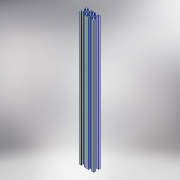
# Autodesk Inventor part: Profile horizontal 20x40x360
Saved by Autodesk Inventor 2017 (Build 210142000, 142)
## iProperties
Company: FABLAB Frenchmakers
Part Number: Profile horizontal 20x40x360
Material: Aluminium
Document SubType Name: Modeling
Designer: FABLAB Frenchmakers
Density: 2.7 g/cm^3
Appearance: Aluminium - Plat(2)
Mass: 278.606 g
Surface Area: 1181.4 cm^2
Volume: 103.187 cm^3
Stock Number: 1420-01-02
Project: 1420 Vauban 3D XL
Catalog Web Link: http://frenchmakers.com/
Autodesk Inventor part; units mm, degrees
ref_plane "YZ Plane" through (0, 0, 0) normal (1, 0, 0) x (0, 1, 0)
ref_plane "XZ Plane" through (0, 0, 0) normal (0, 1, 0) x (-1, 0, 0)
ref_plane "XY Plane" through (0, 0, 0) normal (0, 0, 1) x (1, 0, 0)
sketch "Esquisse1" plane through (0, 0, 0) normal (0, 0, 1) x (1, 0, 0)
  line L0 (-20, -8.5) -> (-20, -3.7)
  arc A0 (-20, -8.5) -> (-18.5, -10) centre (-18.5, -8.5) ccw
  line L1 (-13.7, -10) -> (-18.5, -10)
  arc A1 (-13.7, -10) -> (-13.5, -9.8) centre (-13.7, -9.8) ccw
  line L2 (-13.5, -9.5) -> (-13.5, -9.8)
  line L3 (-13.2, -9.5) -> (-13.5, -9.5)
  arc A2 (-13.2, -9.5) -> (-13, -9.3) centre (-13.2, -9.3) ccw
  line L4 (-13, -9) -> (-13, -9.3)
  arc A3 (-13, -9) -> (-13.5, -8.5) centre (-13.5, -9) ccw
  line L5 (-15.5, -8.5) -> (-13.5, -8.5)
  arc A4 (-16, -8) -> (-15.5, -8.5) centre (-15.5, -8) ccw
  line L6 (-16, -7.2678) -> (-16, -8)
  arc A5 (-15.8536, -6.9142) -> (-16, -7.2678) centre (-15.5, -7.2678) ccw
  line L7 (-13.5858, -4.6464) -> (-15.8536, -6.9142)
  arc A6 (-13.2322, -4.5) -> (-13.5858, -4.6464) centre (-13.2322, -5) ccw
  line L8 (-10.9536, -4.5) -> (-13.2322, -4.5)
  arc A7 (-10.9536, -4.5) -> (-10.8536, -4.4732) centre (-10.9536, -4.3) ccw
  line L9 (-10.1, -4.0381) -> (-10.8536, -4.4732)
  arc A8 (-9.9, -4.0381) -> (-10.1, -4.0381) centre (-10, -4.2113) ccw
  line L10 (-9.1464, -4.4732) -> (-9.9, -4.0381)
  arc A9 (-9.1464, -4.4732) -> (-9.0464, -4.5) centre (-9.0464, -4.3) ccw
  line L11 (-6.7678, -4.5) -> (-9.0464, -4.5)
  arc A10 (-6.4142, -4.6464) -> (-6.7678, -4.5) centre (-6.7678, -5) ccw
  line L12 (-4.1464, -6.9142) -> (-6.4142, -4.6464)
  arc A11 (-4, -7.2678) -> (-4.1464, -6.9142) centre (-4.5, -7.2678) ccw
  line L13 (-4, -8) -> (-4, -7.2678)
  arc A12 (-4.5, -8.5) -> (-4, -8) centre (-4.5, -8) ccw
  line L14 (-6.5, -8.5) -> (-4.5, -8.5)
  arc A13 (-6.5, -8.5) -> (-7, -9) centre (-6.5, -9) ccw
  line L15 (-7, -9.3) -> (-7, -9)
  arc A14 (-7, -9.3) -> (-6.8, -9.5) centre (-6.8, -9.3) ccw
  line L16 (-6.5, -9.5) -> (-6.8, -9.5)
  line L17 (-6.5, -9.8) -> (-6.5, -9.5)
  arc A15 (-6.5, -9.8) -> (-6.3, -10) centre (-6.3, -9.8) ccw
  line L18 (6.3, -10) -> (-6.3, -10)
  arc A16 (6.3, -10) -> (6.5, -9.8) centre (6.3, -9.8) ccw
  line L19 (6.5, -9.5) -> (6.5, -9.8)
  line L20 (6.8, -9.5) -> (6.5, -9.5)
  arc A17 (6.8, -9.5) -> (7, -9.3) centre (6.8, -9.3) ccw
  line L21 (7, -9) -> (7, -9.3)
  arc A18 (7, -9) -> (6.5, -8.5) centre (6.5, -9) ccw
  line L22 (4.5, -8.5) -> (6.5, -8.5)
  arc A19 (4, -8) -> (4.5, -8.5) centre (4.5, -8) ccw
  line L23 (4, -7.2678) -> (4, -8)
  arc A20 (4.1464, -6.9142) -> (4, -7.2678) centre (4.5, -7.2678) ccw
  line L24 (6.4142, -4.6464) -> (4.1464, -6.9142)
  arc A21 (6.7678, -4.5) -> (6.4142, -4.6464) centre (6.7678, -5) ccw
  line L25 (9.0464, -4.5) -> (6.7678, -4.5)
  arc A22 (9.0464, -4.5) -> (9.1464, -4.4732) centre (9.0464, -4.3) ccw
  line L26 (9.9, -4.0381) -> (9.1464, -4.4732)
  arc A23 (10.1, -4.0381) -> (9.9, -4.0381) centre (10, -4.2113) ccw
  line L27 (10.8536, -4.4732) -> (10.1, -4.0381)
  arc A24 (10.8536, -4.4732) -> (10.9536, -4.5) centre (10.9536, -4.3) ccw
  line L28 (13.2322, -4.5) -> (10.9536, -4.5)
  arc A25 (13.5858, -4.6464) -> (13.2322, -4.5) centre (13.2322, -5) ccw
  line L29 (15.8536, -6.9142) -> (13.5858, -4.6464)
  arc A26 (16, -7.2678) -> (15.8536, -6.9142) centre (15.5, -7.2678) ccw
  line L30 (16, -8) -> (16, -7.2678)
  arc A27 (15.5, -8.5) -> (16, -8) centre (15.5, -8) ccw
  line L31 (13.5, -8.5) -> (15.5, -8.5)
  arc A28 (13.5, -8.5) -> (13, -9) centre (13.5, -9) ccw
  line L32 (13, -9.3) -> (13, -9)
  arc A29 (13, -9.3) -> (13.2, -9.5) centre (13.2, -9.3) ccw
  line L33 (13.5, -9.5) -> (13.2, -9.5)
  line L34 (13.5, -9.8) -> (13.5, -9.5)
  arc A30 (13.5, -9.8) -> (13.7, -10) centre (13.7, -9.8) ccw
  line L35 (18.5, -10) -> (13.7, -10)
  arc A31 (18.5, -10) -> (20, -8.5) centre (18.5, -8.5) ccw
  line L36 (20, -3.7) -> (20, -8.5)
  arc A32 (20, -3.7) -> (19.8, -3.5) centre (19.8, -3.7) ccw
  line L37 (19.5, -3.5) -> (19.8, -3.5)
  line L38 (19.5, -3.2) -> (19.5, -3.5)
  arc A33 (19.5, -3.2) -> (19.3, -3) centre (19.3, -3.2) ccw
  line L39 (19, -3) -> (19.3, -3)
  arc A34 (19, -3) -> (18.5, -3.5) centre (19, -3.5) ccw
  line L40 (18.5, -5.5) -> (18.5, -3.5)
  arc A35 (18, -6) -> (18.5, -5.5) centre (18, -5.5) ccw
  line L41 (17.2678, -6) -> (18, -6)
  arc A36 (16.9142, -5.8536) -> (17.2678, -6) centre (17.2678, -5.5) ccw
  line L42 (14.6464, -3.5858) -> (16.9142, -5.8536)
  arc A37 (14.5, -3.2322) -> (14.6464, -3.5858) centre (15, -3.2322) ccw
  line L43 (14.5, -0.9536) -> (14.5, -3.2322)
  arc A38 (14.5, -0.9536) -> (14.4732, -0.8536) centre (14.3, -0.9536) ccw
  line L44 (14.0381, -0.1) -> (14.4732, -0.8536)
  arc A39 (14.0381, 0.1) -> (14.0381, -0.1) centre (14.2113, 0) ccw
  line L45 (14.4732, 0.8536) -> (14.0381, 0.1)
  arc A40 (14.4732, 0.8536) -> (14.5, 0.9536) centre (14.3, 0.9536) ccw
  line L46 (14.5, 3.2322) -> (14.5, 0.9536)
  arc A41 (14.6464, 3.5858) -> (14.5, 3.2322) centre (15, 3.2322) ccw
  line L47 (16.9142, 5.8536) -> (14.6464, 3.5858)
  arc A42 (17.2678, 6) -> (16.9142, 5.8536) centre (17.2678, 5.5) ccw
  line L48 (18, 6) -> (17.2678, 6)
  arc A43 (18.5, 5.5) -> (18, 6) centre (18, 5.5) ccw
  line L49 (18.5, 3.5) -> (18.5, 5.5)
  arc A44 (18.5, 3.5) -> (19, 3) centre (19, 3.5) ccw
  line L50 (19.3, 3) -> (19, 3)
  arc A45 (19.3, 3) -> (19.5, 3.2) centre (19.3, 3.2) ccw
  line L51 (19.5, 3.5) -> (19.5, 3.2)
  line L52 (19.8, 3.5) -> (19.5, 3.5)
  arc A46 (19.8, 3.5) -> (20, 3.7) centre (19.8, 3.7) ccw
  line L53 (20, 8.5) -> (20, 3.7)
  arc A47 (20, 8.5) -> (18.5, 10) centre (18.5, 8.5) ccw
  line L54 (13.7, 10) -> (18.5, 10)
  arc A48 (13.7, 10) -> (13.5, 9.8) centre (13.7, 9.8) ccw
  line L55 (13.5, 9.5) -> (13.5, 9.8)
  line L56 (13.2, 9.5) -> (13.5, 9.5)
  arc A49 (13.2, 9.5) -> (13, 9.3) centre (13.2, 9.3) ccw
  line L57 (13, 9) -> (13, 9.3)
  arc A50 (13, 9) -> (13.5, 8.5) centre (13.5, 9) ccw
  line L58 (15.5, 8.5) -> (13.5, 8.5)
  arc A51 (16, 8) -> (15.5, 8.5) centre (15.5, 8) ccw
  line L59 (16, 7.2678) -> (16, 8)
  arc A52 (15.8536, 6.9142) -> (16, 7.2678) centre (15.5, 7.2678) ccw
  line L60 (13.5858, 4.6464) -> (15.8536, 6.9142)
  arc A53 (13.2322, 4.5) -> (13.5858, 4.6464) centre (13.2322, 5) ccw
  line L61 (10.9536, 4.5) -> (13.2322, 4.5)
  arc A54 (10.9536, 4.5) -> (10.8536, 4.4732) centre (10.9536, 4.3) ccw
  line L62 (10.1, 4.0381) -> (10.8536, 4.4732)
  arc A55 (9.9, 4.0381) -> (10.1, 4.0381) centre (10, 4.2113) ccw
  line L63 (9.1464, 4.4732) -> (9.9, 4.0381)
  arc A56 (9.1464, 4.4732) -> (9.0464, 4.5) centre (9.0464, 4.3) ccw
  line L64 (6.7678, 4.5) -> (9.0464, 4.5)
  arc A57 (6.4142, 4.6464) -> (6.7678, 4.5) centre (6.7678, 5) ccw
  line L65 (4.1464, 6.9142) -> (6.4142, 4.6464)
  arc A58 (4, 7.2678) -> (4.1464, 6.9142) centre (4.5, 7.2678) ccw
  line L66 (4, 8) -> (4, 7.2678)
  arc A59 (4.5, 8.5) -> (4, 8) centre (4.5, 8) ccw
  line L67 (6.5, 8.5) -> (4.5, 8.5)
  arc A60 (6.5, 8.5) -> (7, 9) centre (6.5, 9) ccw
  line L68 (7, 9.3) -> (7, 9)
  arc A61 (7, 9.3) -> (6.8, 9.5) centre (6.8, 9.3) ccw
  line L69 (6.5, 9.5) -> (6.8, 9.5)
  line L70 (6.5, 9.8) -> (6.5, 9.5)
  arc A62 (6.5, 9.8) -> (6.3, 10) centre (6.3, 9.8) ccw
  line L71 (-6.3, 10) -> (6.3, 10)
  arc A63 (-6.3, 10) -> (-6.5, 9.8) centre (-6.3, 9.8) ccw
  line L72 (-6.5, 9.5) -> (-6.5, 9.8)
  line L73 (-6.8, 9.5) -> (-6.5, 9.5)
  arc A64 (-6.8, 9.5) -> (-7, 9.3) centre (-6.8, 9.3) ccw
  line L74 (-7, 9) -> (-7, 9.3)
  arc A65 (-7, 9) -> (-6.5, 8.5) centre (-6.5, 9) ccw
  line L75 (-4.5, 8.5) -> (-6.5, 8.5)
  arc A66 (-4, 8) -> (-4.5, 8.5) centre (-4.5, 8) ccw
  line L76 (-4, 7.2678) -> (-4, 8)
  arc A67 (-4.1464, 6.9142) -> (-4, 7.2678) centre (-4.5, 7.2678) ccw
  line L77 (-6.4142, 4.6464) -> (-4.1464, 6.9142)
  arc A68 (-6.7678, 4.5) -> (-6.4142, 4.6464) centre (-6.7678, 5) ccw
  line L78 (-9.0464, 4.5) -> (-6.7678, 4.5)
  arc A69 (-9.0464, 4.5) -> (-9.1464, 4.4732) centre (-9.0464, 4.3) ccw
  line L79 (-9.9, 4.0381) -> (-9.1464, 4.4732)
  arc A70 (-10.1, 4.0381) -> (-9.9, 4.0381) centre (-10, 4.2113) ccw
  line L80 (-10.8536, 4.4732) -> (-10.1, 4.0381)
  arc A71 (-10.8536, 4.4732) -> (-10.9536, 4.5) centre (-10.9536, 4.3) ccw
  line L81 (-13.2322, 4.5) -> (-10.9536, 4.5)
  arc A72 (-13.5858, 4.6464) -> (-13.2322, 4.5) centre (-13.2322, 5) ccw
  line L82 (-15.8536, 6.9142) -> (-13.5858, 4.6464)
  arc A73 (-16, 7.2678) -> (-15.8536, 6.9142) centre (-15.5, 7.2678) ccw
  line L83 (-16, 8) -> (-16, 7.2678)
  arc A74 (-15.5, 8.5) -> (-16, 8) centre (-15.5, 8) ccw
  line L84 (-13.5, 8.5) -> (-15.5, 8.5)
  arc A75 (-13.5, 8.5) -> (-13, 9) centre (-13.5, 9) ccw
  line L85 (-13, 9.3) -> (-13, 9)
  arc A76 (-13, 9.3) -> (-13.2, 9.5) centre (-13.2, 9.3) ccw
  line L86 (-13.5, 9.5) -> (-13.2, 9.5)
  line L87 (-13.5, 9.8) -> (-13.5, 9.5)
  arc A77 (-13.5, 9.8) -> (-13.7, 10) centre (-13.7, 9.8) ccw
  line L88 (-18.5, 10) -> (-13.7, 10)
  arc A78 (-18.5, 10) -> (-20, 8.5) centre (-18.5, 8.5) ccw
  line L89 (-20, 3.7) -> (-20, 8.5)
  arc A79 (-20, 3.7) -> (-19.8, 3.5) centre (-19.8, 3.7) ccw
  line L90 (-19.5, 3.5) -> (-19.8, 3.5)
  line L91 (-19.5, 3.2) -> (-19.5, 3.5)
  arc A80 (-19.5, 3.2) -> (-19.3, 3) centre (-19.3, 3.2) ccw
  line L92 (-19, 3) -> (-19.3, 3)
  arc A81 (-19, 3) -> (-18.5, 3.5) centre (-19, 3.5) ccw
  line L93 (-18.5, 5.5) -> (-18.5, 3.5)
  arc A82 (-18, 6) -> (-18.5, 5.5) centre (-18, 5.5) ccw
  line L94 (-17.2678, 6) -> (-18, 6)
  arc A83 (-16.9142, 5.8536) -> (-17.2678, 6) centre (-17.2678, 5.5) ccw
  line L95 (-14.6464, 3.5858) -> (-16.9142, 5.8536)
  arc A84 (-14.5, 3.2322) -> (-14.6464, 3.5858) centre (-15, 3.2322) ccw
  line L96 (-14.5, 0.9536) -> (-14.5, 3.2322)
  arc A85 (-14.5, 0.9536) -> (-14.4732, 0.8536) centre (-14.3, 0.9536) ccw
  line L97 (-14.0381, 0.1) -> (-14.4732, 0.8536)
  arc A86 (-14.0381, -0.1) -> (-14.0381, 0.1) centre (-14.2113, 0) ccw
  line L98 (-14.4732, -0.8536) -> (-14.0381, -0.1)
  arc A87 (-14.4732, -0.8536) -> (-14.5, -0.9536) centre (-14.3, -0.9536) ccw
  line L99 (-14.5, -3.2322) -> (-14.5, -0.9536)
  arc A88 (-14.6464, -3.5858) -> (-14.5, -3.2322) centre (-15, -3.2322) ccw
  line L100 (-16.9142, -5.8536) -> (-14.6464, -3.5858)
  arc A89 (-17.2678, -6) -> (-16.9142, -5.8536) centre (-17.2678, -5.5) ccw
  line L101 (-18, -6) -> (-17.2678, -6)
  arc A90 (-18.5, -5.5) -> (-18, -6) centre (-18, -5.5) ccw
  line L102 (-18.5, -3.5) -> (-18.5, -5.5)
  arc A91 (-18.5, -3.5) -> (-19, -3) centre (-19, -3.5) ccw
  line L103 (-19.3, -3) -> (-19, -3)
  arc A92 (-19.3, -3) -> (-19.5, -3.2) centre (-19.3, -3.2) ccw
  line L104 (-19.5, -3.5) -> (-19.5, -3.2)
  line L105 (-19.8, -3.5) -> (-19.5, -3.5)
  arc A93 (-19.8, -3.5) -> (-20, -3.7) centre (-19.8, -3.7) ccw
  arc A94 (-2.5, -6.6464) -> (-2.6464, -6.2929) centre (-3, -6.6464) ccw
  line L106 (-2.6464, -6.2929) -> (-5.3536, -3.5858)
  arc A95 (-5.5, -3.2322) -> (-5.3536, -3.5858) centre (-5, -3.2322) ccw
  line L107 (-5.5, -3.2322) -> (-5.5, -0.9536)
  arc A96 (-5.5, -0.9536) -> (-5.5268, -0.8536) centre (-5.7, -0.9536) ccw
  line L108 (-5.5268, -0.8536) -> (-5.9619, -0.1)
  arc A97 (-5.9619, 0.1) -> (-5.9619, -0.1) centre (-5.7887, 0) ccw
  line L109 (-5.9619, 0.1) -> (-5.5268, 0.8536)
  arc A98 (-5.5268, 0.8536) -> (-5.5, 0.9536) centre (-5.7, 0.9536) ccw
  line L110 (-5.5, 0.9536) -> (-5.5, 3.2322)
  arc A99 (-5.3536, 3.5858) -> (-5.5, 3.2322) centre (-5, 3.2322) ccw
  line L111 (-5.3536, 3.5858) -> (-2.6464, 6.2929)
  arc A100 (-2.6464, 6.2929) -> (-2.5, 6.6464) centre (-3, 6.6464) ccw
  line L112 (-2.5, 6.6464) -> (-2.5, 8)
  arc A101 (-2, 8.5) -> (-2.5, 8) centre (-2, 8) ccw
  line L113 (-2, 8.5) -> (2, 8.5)
  arc A102 (2.5, 8) -> (2, 8.5) centre (2, 8) ccw
  line L114 (2.5, 8) -> (2.5, 6.6464)
  arc A103 (2.5, 6.6464) -> (2.6464, 6.2929) centre (3, 6.6464) ccw
  line L115 (2.6464, 6.2929) -> (5.3536, 3.5858)
  arc A104 (5.5, 3.2322) -> (5.3536, 3.5858) centre (5, 3.2322) ccw
  line L116 (5.5, 3.2322) -> (5.5, 0.9536)
  arc A105 (5.5, 0.9536) -> (5.5268, 0.8536) centre (5.7, 0.9536) ccw
  line L117 (5.5268, 0.8536) -> (5.9619, 0.1)
  arc A106 (5.9619, -0.1) -> (5.9619, 0.1) centre (5.7887, 0) ccw
  line L118 (5.9619, -0.1) -> (5.5268, -0.8536)
  arc A107 (5.5268, -0.8536) -> (5.5, -0.9536) centre (5.7, -0.9536) ccw
  line L119 (5.5, -0.9536) -> (5.5, -3.2322)
  arc A108 (5.3536, -3.5858) -> (5.5, -3.2322) centre (5, -3.2322) ccw
  line L120 (5.3536, -3.5858) -> (2.6464, -6.2929)
  arc A109 (2.6464, -6.2929) -> (2.5, -6.6464) centre (3, -6.6464) ccw
  line L121 (2.5, -6.6464) -> (2.5, -8)
  arc A110 (2, -8.5) -> (2.5, -8) centre (2, -8) ccw
  line L122 (2, -8.5) -> (-2, -8.5)
  arc A111 (-2.5, -8) -> (-2, -8.5) centre (-2, -8) ccw
  line L123 (-2.5, -8) -> (-2.5, -6.6464)
  arc A112 (-12.9896, -1.9139) -> (-11.9099, -2.9922) centre (-10, 0) ccw
  line L124 (-12.9896, -1.9139) -> (-12.4453, -1.2582)
  arc A113 (-12.4453, 1.2582) -> (-12.4453, -1.2582) centre (-10, 0) ccw
  line L125 (-12.4453, 1.2582) -> (-12.9896, 1.9139)
  arc A114 (-11.9099, 2.9922) -> (-12.9896, 1.9139) centre (-10, 0) ccw
  line L126 (-11.9099, 2.9922) -> (-11.2582, 2.4453)
  arc A115 (-8.7418, 2.4453) -> (-11.2582, 2.4453) centre (-10, 0) ccw
  line L127 (-8.7418, 2.4453) -> (-8.0901, 2.9922)
  arc A116 (-7.0104, 1.9139) -> (-8.0901, 2.9922) centre (-10, 0) ccw
  line L128 (-7.0104, 1.9139) -> (-7.5547, 1.2582)
  arc A117 (-7.5547, -1.2582) -> (-7.5547, 1.2582) centre (-10, 0) ccw
  line L129 (-7.5547, -1.2582) -> (-7.0104, -1.9139)
  arc A118 (-8.0901, -2.9922) -> (-7.0104, -1.9139) centre (-10, 0) ccw
  line L130 (-8.0901, -2.9922) -> (-8.7418, -2.4453)
  arc A119 (-11.2582, -2.4453) -> (-8.7418, -2.4453) centre (-10, 0) ccw
  line L131 (-11.2582, -2.4453) -> (-11.9099, -2.9922)
  arc A120 (7.0104, -1.9139) -> (8.0901, -2.9922) centre (10, 0) ccw
  line L132 (7.0104, -1.9139) -> (7.5547, -1.2582)
  arc A121 (7.5547, 1.2582) -> (7.5547, -1.2582) centre (10, 0) ccw
  line L133 (7.5547, 1.2582) -> (7.0104, 1.9139)
  arc A122 (8.0901, 2.9922) -> (7.0104, 1.9139) centre (10, 0) ccw
  line L134 (8.0901, 2.9922) -> (8.7418, 2.4453)
  arc A123 (11.2582, 2.4453) -> (8.7418, 2.4453) centre (10, 0) ccw
  line L135 (11.2582, 2.4453) -> (11.9099, 2.9922)
  arc A124 (12.9896, 1.9139) -> (11.9099, 2.9922) centre (10, 0) ccw
  line L136 (12.9896, 1.9139) -> (12.4453, 1.2582)
  arc A125 (12.4453, -1.2582) -> (12.4453, 1.2582) centre (10, 0) ccw
  line L137 (12.4453, -1.2582) -> (12.9896, -1.9139)
  arc A126 (11.9099, -2.9922) -> (12.9896, -1.9139) centre (10, 0) ccw
  line L138 (11.9099, -2.9922) -> (11.2582, -2.4453)
  arc A127 (8.7418, -2.4453) -> (11.2582, -2.4453) centre (10, 0) ccw
  line L139 (8.7418, -2.4453) -> (8.0901, -2.9922)
  line L140 (-10, 0) -> (10, 0) construction
  line L141 (0, -8.5) -> (0, 8.5) construction
  point P0 (0, 0)
  point P1 (-6.3, -10)
  point P2 (0, 0)
  constraints: 284 end point, 256 point on circle, 128 centre point, 4 midpoint, 1 horizontal
extrude "Extrusion1" add sketch "Esquisse1" along normal mid plane 360
sketch "Esquisse2" plane through (-6.3, 10, 180) normal (0, 1, 0) x (1, 0, 0)
  line L0 (3.0705, 11.9482) -> (2.9892, 12.1296)
  line L1 (3.0771, 11.9001) -> (3.0705, 11.9482)
  line L2 (3.078, 11.8916) -> (3.0771, 11.9001)
  line L3 (3.0799, 11.7602) -> (3.078, 11.8916)
  line L4 (3.0828, 11.4249) -> (3.0799, 11.7602)
  line L5 (3.5457, 12.2317) -> (3.3681, 11.8453)
  line L6 (3.3029, 11.5184) -> (3.3085, 11.4683)
  line L7 (3.3681, 11.8453) -> (3.3029, 11.5184)
  line L8 (3.4162, 11.6251) -> (3.6921, 12.0739)
  line L9 (3.3728, 11.5316) -> (3.4162, 11.6251)
  line L10 (3.3085, 11.4683) -> (3.3161, 11.4079)
  line L11 (3.6222, 11.7092) -> (3.5617, 11.5873)
  line L12 (3.5617, 11.5873) -> (3.5287, 11.5193)
  line L13 (3.3161, 11.4079) -> (3.3728, 11.5316)
  line L14 (2.9892, 12.1296) -> (2.8617, 12.208)
  line L15 (2.8617, 12.208) -> (2.8324, 12.2043)
  line L16 (2.8324, 12.2043) -> (2.703, 12.123)
  line L17 (2.6435, 8.8202) -> (2.6567, 8.7891)
  line L18 (2.6567, 8.7891) -> (2.7984, 8.6266)
  line L19 (2.7984, 8.6266) -> (2.8447, 8.6266)
  line L20 (2.8447, 8.6266) -> (2.8985, 8.6266)
  line L21 (2.8985, 8.6266) -> (3.0469, 8.808)
  line L22 (3.5287, 11.5193) -> (3.3189, 10.8004)
  line L23 (3.3189, 10.8004) -> (3.3076, 10.7135)
  line L24 (3.3076, 10.7135) -> (3.301, 10.6643)
  line L25 (3.301, 10.6643) -> (3.2887, 10.2902)
  line L26 (2.4167, 11.1121) -> (2.4148, 11.5467)
  line L27 (3.0837, 10.9468) -> (3.0828, 11.4249)
  line L28 (2.6198, 11.3729) -> (2.6189, 10.6483)
  line L29 (2.6189, 10.6483) -> (2.6189, 10.4064)
  line L30 (3.0837, 10.5179) -> (3.0837, 10.9468)
  line L31 (3.0837, 10.3743) -> (3.0837, 10.5179)
  line L32 (2.6265, 11.85) -> (2.6198, 11.3729)
  line L33 (2.703, 12.123) -> (2.6907, 12.106)
  line L34 (2.6907, 12.106) -> (2.6794, 12.089)
  line L35 (2.6794, 12.089) -> (2.6472, 12.0314)
  line L36 (2.6472, 12.0314) -> (2.6265, 11.85)
  line L37 (2.1418, 12.0777) -> (2.0351, 11.9945)
  line L38 (2.4148, 11.5467) -> (2.4111, 11.7678)
  line L39 (2.4111, 11.7678) -> (2.4063, 11.8377)
  line L40 (2.4063, 11.8377) -> (2.4026, 11.849)
  line L41 (2.4026, 11.849) -> (2.3931, 11.8859)
  line L42 (1.9576, 11.7414) -> (1.95, 11.3219)
  line L43 (1.9793, 11.9038) -> (1.9576, 11.7414)
  line L44 (2.3931, 11.8859) -> (2.2344, 12.0777)
  line L45 (2.0114, 11.9596) -> (1.9793, 11.9038)
  line L46 (2.0228, 11.9766) -> (2.0114, 11.9596)
  line L47 (2.0351, 11.9945) -> (2.0228, 11.9766)
  line L48 (2.2344, 12.0777) -> (2.1805, 12.0777)
  line L49 (2.1805, 12.0777) -> (2.1418, 12.0777)
  line L50 (1.7025, 11.1159) -> (1.6978, 11.1235)
  line L51 (1.95, 11.3219) -> (1.9472, 10.688)
  line L52 (2.4167, 10.5708) -> (2.4167, 11.1121)
  line L53 (2.4158, 10.3904) -> (2.4167, 10.5708)
  line L54 (1.9472, 10.688) -> (1.9462, 10.4764)
  line L55 (2.3742, 8.9034) -> (2.3884, 8.9346)
  line L56 (2.1815, 8.756) -> (2.2334, 8.756)
  line L57 (2.2334, 8.756) -> (2.3742, 8.9034)
  line L58 (2.1456, 8.756) -> (2.1815, 8.756)
  line L59 (2.0351, 8.8373) -> (2.1456, 8.756)
  line L60 (1.9623, 9.0092) -> (2.0351, 8.8373)
  line L61 (1.9538, 9.0687) -> (1.9623, 9.0092)
  line L62 (1.9481, 9.4532) -> (1.9538, 9.0687)
  line L63 (1.6798, 9.6847) -> (1.6931, 9.7045)
  line L64 (1.6931, 9.7045) -> (1.7176, 9.7413)
  line L65 (1.4503, 9.6025) -> (1.6798, 9.6847)
  line L66 (1.4229, 9.6082) -> (1.4503, 9.6025)
  line L67 (1.3974, 9.6138) -> (1.4229, 9.6082)
  line L68 (1.3048, 9.6696) -> (1.3974, 9.6138)
  line L69 (1.2018, 9.8254) -> (1.3048, 9.6696)
  line L70 (1.1716, 9.8793) -> (1.2018, 9.8254)
  line L71 (1.1376, 9.9426) -> (1.1716, 9.8793)
  line L72 (1.0355, 10.1334) -> (1.1376, 9.9426)
  line L73 (0.9874, 10.2458) -> (1.0355, 10.1334)
  line L74 (0.9788, 10.2704) -> (0.9874, 10.2458)
  line L75 (0.9666, 10.3091) -> (0.9788, 10.2704)
  line L76 (0.9581, 10.4877) -> (0.9666, 10.3091)
  line L77 (1.6978, 11.1235) -> (1.6874, 11.1424)
  line L78 (1.7148, 10.9978) -> (1.7025, 11.1159)
  line L79 (1.6874, 11.1424) -> (1.5315, 11.2293)
  line L80 (1.5315, 11.2293) -> (1.4796, 11.2293)
  line L81 (1.4796, 11.2293) -> (1.4333, 11.2293)
  line L82 (1.4333, 11.2293) -> (1.3029, 11.1736)
  line L83 (1.3029, 11.1736) -> (1.2887, 11.1575)
  line L84 (1.7176, 10.5614) -> (1.7148, 10.9978)
  line L85 (1.7176, 10.4159) -> (1.7176, 10.5614)
  line L86 (1.2887, 11.1575) -> (1.1971, 11.0045)
  line L87 (1.1971, 11.0045) -> (1.079, 10.79)
  line L88 (1.079, 10.79) -> (1.0591, 10.7522)
  line L89 (1.0591, 10.7522) -> (1.0308, 10.6984)
  line L90 (1.0308, 10.6984) -> (0.9581, 10.4877)
  line L91 (3.2887, 10.2902) -> (3.3019, 9.9057)
  line L92 (3.0469, 8.808) -> (3.0582, 8.842)
  line L93 (2.6189, 8.8807) -> (2.6435, 8.8202)
  line L94 (3.0582, 8.842) -> (3.0818, 8.9128)
  line L95 (2.3884, 8.9346) -> (2.4139, 8.9884)
  line L96 (3.3397, 9.5874) -> (3.5523, 8.808)
  line L97 (3.3076, 9.851) -> (3.3397, 9.5874)
  line L98 (3.3019, 9.9057) -> (3.3076, 9.851)
  line L99 (3.0818, 8.9128) -> (3.0837, 10.3743)
  line L100 (2.6189, 10.4064) -> (2.6189, 8.8807)
  line L101 (2.4139, 8.9884) -> (2.4158, 10.3904)
  line L102 (1.9462, 10.2543) -> (1.9481, 9.4532)
  line L103 (1.9462, 10.4764) -> (1.9462, 10.2543)
  line L104 (1.7176, 9.7413) -> (1.7176, 10.4159)
  line L105 (9.5154, 12.2184) -> (9.4701, 12.2883)
  line L106 (9.5655, 12.1438) -> (9.5154, 12.2184)
  line L107 (9.7847, 11.6988) -> (9.5655, 12.1438)
  line L108 (9.95, 11.1915) -> (9.7847, 11.6988)
  line L109 (9.9727, 11.0848) -> (9.95, 11.1915)
  line L110 (9.9783, 11.0573) -> (9.9727, 11.0848)
  line L111 (9.4701, 12.2883) -> (9.5532, 12.3998)
  line L112 (6.8579, 14.5973) -> (6.9004, 14.5056)
  line L113 (7.267, 14.6936) -> (7.0431, 14.6965)
  line L114 (6.9004, 14.5056) -> (6.9609, 14.1013)
  line L115 (7.2925, 14.208) -> (7.267, 14.6936)
  line L116 (7.2962, 14.1419) -> (7.2925, 14.208)
  line L117 (6.9609, 14.1013) -> (6.8569, 13.6913)
  line L118 (7.3114, 13.8651) -> (7.2962, 14.1419)
  line L119 (7.3218, 13.7196) -> (7.3114, 13.8651)
  line L120 (7.4663, 13.6809) -> (7.3218, 13.7196)
  line L121 (7.489, 13.6752) -> (7.4663, 13.6809)
  line L122 (7.5381, 13.6629) -> (7.489, 13.6752)
  line L123 (8.0152, 13.4995) -> (7.5381, 13.6629)
  line L124 (8.0558, 13.4806) -> (8.0152, 13.4995)
  line L125 (8.087, 13.4674) -> (8.0558, 13.4806)
  line L126 (7.0431, 14.6965) -> (7.0128, 14.6974)
  line L127 (6.2703, 13.4003) -> (6.3393, 13.4806)
  line L128 (6.2363, 13.3606) -> (6.2703, 13.4003)
  line L129 (5.9774, 13.1036) -> (6.2363, 13.3606)
  line L130 (6.2589, 12.5623) -> (6.4413, 12.5973)
  line L131 (6.206, 12.5519) -> (6.2589, 12.5623)
  line L132 (6.4479, 13.1206) -> (5.933, 12.6275)
  line L133 (5.933, 12.6275) -> (5.7894, 12.5047)
  line L134 (5.5731, 12.7418) -> (5.9774, 13.1036)
  line L135 (5.7894, 12.5047) -> (5.7299, 12.4546)
  line L136 (5.6354, 12.3375) -> (6.206, 12.5519)
  line L137 (5.5806, 12.3063) -> (5.6354, 12.3375)
  line L138 (5.7299, 12.4546) -> (5.5523, 12.2997)
  line L139 (4.668, 7.099) -> (5.2764, 6.6172)
  line L140 (3.5523, 8.808) -> (4.0124, 7.8802)
  line L141 (4.0124, 7.8802) -> (4.668, 7.099)
  line L142 (6.4167, 6.1183) -> (6.5065, 6.0938)
  line L143 (6.5065, 6.0938) -> (6.5414, 6.0852)
  line L144 (6.5414, 6.0852) -> (6.7852, 6.0305)
  line L145 (6.9127, 6.0494) -> (6.8144, 6.1221)
  line L146 (6.9221, 6.0428) -> (6.9127, 6.0494)
  line L147 (6.7852, 6.0305) -> (6.9675, 5.9965)
  line L148 (6.9675, 5.9965) -> (6.9221, 6.0428)
  line L149 (4.3685, 11.0942) -> (4.3685, 11.2208)
  line L150 (4.3685, 11.2208) -> (4.3685, 11.2973)
  line L151 (4.3685, 11.2973) -> (4.4035, 11.524)
  line L152 (4.4035, 11.524) -> (4.4999, 11.7177)
  line L153 (5.2641, 11.5127) -> (5.2084, 11.1405)
  line L154 (4.4592, 10.7116) -> (4.3685, 11.0942)
  line L155 (5.2084, 11.1405) -> (5.2018, 11.0262)
  line L156 (5.2018, 11.0262) -> (5.1989, 10.9676)
  line L157 (5.1989, 10.9676) -> (5.1763, 10.7617)
  line L158 (4.6444, 10.4471) -> (4.4592, 10.7116)
  line L159 (5.1763, 10.7617) -> (5.1375, 10.6275)
  line L160 (4.6916, 10.4254) -> (4.6444, 10.4471)
  line L161 (4.7304, 10.4093) -> (4.6916, 10.4254)
  line L162 (5.1375, 10.6275) -> (5.1262, 10.6039)
  line L163 (5.1262, 10.6039) -> (5.1064, 10.5633)
  line L164 (5.1064, 10.5633) -> (4.9363, 10.4282)
  line L165 (4.9363, 10.4282) -> (4.7304, 10.4093)
  line L166 (4.4999, 11.7177) -> (4.531, 11.7584)
  line L167 (4.531, 11.7584) -> (4.5631, 11.7999)
  line L168 (4.5631, 11.7999) -> (4.6642, 11.918)
  line L169 (4.6642, 11.918) -> (4.8381, 12.0937)
  line L170 (4.0464, 12.3016) -> (3.6222, 11.7092)
  line L171 (4.0681, 12.5207) -> (4.1607, 12.6133)
  line L172 (3.5948, 12.311) -> (3.5457, 12.2317)
  line L173 (4.1607, 12.6133) -> (4.2344, 12.687)
  line L174 (3.6921, 12.0739) -> (4.0681, 12.5207)
  line L175 (3.6723, 12.4338) -> (3.5948, 12.311)
  line L176 (4.6878, 12.927) -> (4.0464, 12.3016)
  line L177 (4.258, 13.1471) -> (3.6723, 12.4338)
  line L178 (5.8791, 9.9445) -> (5.9774, 10.4773)
  line L179 (5.8007, 9.4551) -> (5.8791, 9.9445)
  line L180 (5.7601, 9.0857) -> (5.8007, 9.4551)
  line L181 (5.7459, 8.8193) -> (5.7601, 9.0857)
  line L182 (5.9774, 10.4773) -> (6.0105, 10.654)
  line L183 (6.087, 11.7328) -> (6.0813, 11.7498)
  line L184 (6.0813, 11.7498) -> (6.0133, 11.8623)
  line L185 (6.0133, 11.8623) -> (5.9887, 11.8878)
  line L186 (5.3841, 11.7338) -> (5.2641, 11.5127)
  line L187 (5.9887, 11.8878) -> (5.8839, 11.9501)
  line L188 (5.4219, 11.7706) -> (5.3841, 11.7338)
  line L189 (5.4417, 11.7905) -> (5.4219, 11.7706)
  line L190 (5.8839, 11.9501) -> (5.8499, 11.9596)
  line L191 (5.8499, 11.9596) -> (5.745, 11.9549)
  line L192 (5.745, 11.9549) -> (5.728, 11.9482)
  line L193 (5.728, 11.9482) -> (5.6921, 11.936)
  line L194 (5.6921, 11.936) -> (5.4417, 11.7905)
  line L195 (6.0331, 10.7711) -> (6.0936, 11.1396)
  line L196 (6.0936, 11.1396) -> (6.1116, 11.3899)
  line L197 (6.1116, 11.3899) -> (6.1116, 11.4475)
  line L198 (6.1116, 11.4475) -> (6.1116, 11.4938)
  line L199 (6.1116, 11.4938) -> (6.1087, 11.6337)
  line L200 (6.1087, 11.6337) -> (6.0936, 11.7149)
  line L201 (6.0936, 11.7149) -> (6.087, 11.7328)
  line L202 (6.0105, 10.654) -> (6.0331, 10.7711)
  line L203 (5.5523, 12.2997) -> (5.5806, 12.3063)
  line L204 (4.8381, 12.0937) -> (5.0922, 12.3261)
  line L205 (5.0922, 12.3261) -> (5.3728, 12.5699)
  line L206 (5.3728, 12.5699) -> (5.4663, 12.6502)
  line L207 (5.4663, 12.6502) -> (5.5731, 12.7418)
  line L208 (5.5088, 13.5722) -> (5.1243, 13.2784)
  line L209 (5.1243, 13.2784) -> (4.8929, 13.0961)
  line L210 (4.8929, 13.0961) -> (4.856, 13.0659)
  line L211 (4.856, 13.0659) -> (4.6878, 12.927)
  line L212 (5.2065, 13.4957) -> (5.3057, 13.5713)
  line L213 (5.0657, 13.389) -> (5.2065, 13.4957)
  line L214 (5.0846, 13.9633) -> (4.258, 13.1471)
  line L215 (4.582, 13.0035) -> (5.0657, 13.389)
  line L216 (4.2344, 12.687) -> (4.582, 13.0035)
  line L217 (5.744, 8.7295) -> (5.7459, 8.8193)
  line L218 (5.7412, 8.5784) -> (5.744, 8.7295)
  line L219 (5.7951, 7.9076) -> (5.7412, 8.5784)
  line L220 (5.9491, 7.3172) -> (5.7951, 7.9076)
  line L221 (5.9954, 7.2048) -> (5.9491, 7.3172)
  line L222 (6.0426, 7.0942) -> (5.9954, 7.2048)
  line L223 (6.0785, 8.3139) -> (6.0823, 8.1967)
  line L224 (6.104, 8.3139) -> (6.0785, 8.3139)
  line L225 (6.0823, 8.1967) -> (6.1068, 8.0021)
  line L226 (6.1068, 8.0021) -> (6.1125, 7.9634)
  line L227 (6.1125, 7.9634) -> (6.1437, 7.7829)
  line L228 (6.1956, 8.2874) -> (6.104, 8.3139)
  line L229 (6.2892, 8.2657) -> (6.1956, 8.2874)
  line L230 (6.1437, 7.7829) -> (6.4545, 7.0149)
  line L231 (5.7308, 13.7394) -> (5.6222, 13.6582)
  line L232 (5.6222, 13.6582) -> (5.5088, 13.5722)
  line L233 (5.5211, 14.346) -> (5.3407, 14.191)
  line L234 (5.3407, 14.191) -> (5.2812, 14.1381)
  line L235 (5.5995, 13.8018) -> (5.8593, 14.0191)
  line L236 (5.2812, 14.1381) -> (5.0846, 13.9633)
  line L237 (5.3057, 13.5713) -> (5.5995, 13.8018)
  line L238 (7.3652, 8.3413) -> (7.2707, 8.311)
  line L239 (7.2707, 8.311) -> (6.2892, 8.2657)
  line L240 (6.1956, 14.6842) -> (6.1843, 14.7116)
  line L241 (6.1843, 14.7116) -> (6.1267, 14.8391)
  line L242 (6.1267, 14.8391) -> (6.1087, 14.8391)
  line L243 (6.1087, 14.8391) -> (6.0851, 14.8391)
  line L244 (6.0851, 14.8391) -> (6.0124, 14.7626)
  line L245 (6.0124, 14.7626) -> (5.7903, 14.5765)
  line L246 (5.7903, 14.5765) -> (5.5211, 14.346)
  line L247 (6.1456, 14.3564) -> (6.1956, 14.6842)
  line L248 (6.6425, 14.1655) -> (6.6359, 14.2269)
  line L249 (6.6359, 14.2269) -> (6.634, 14.2449)
  line L250 (6.634, 14.2449) -> (6.5962, 14.4178)
  line L251 (6.5962, 14.4178) -> (6.5603, 14.4178)
  line L252 (6.5603, 14.4178) -> (6.5027, 14.3526)
  line L253 (6.5027, 14.3526) -> (6.4517, 14.3072)
  line L254 (6.1257, 14.3233) -> (6.1456, 14.3564)
  line L255 (6.1031, 14.2864) -> (6.1257, 14.3233)
  line L256 (6.4517, 14.3072) -> (6.1597, 14.071)
  line L257 (6.0218, 14.1825) -> (6.1031, 14.2864)
  line L258 (5.8593, 14.0191) -> (6.0218, 14.1825)
  line L259 (6.1597, 14.071) -> (5.7308, 13.7394)
  line L260 (6.3393, 13.4806) -> (6.566, 13.8424)
  line L261 (6.566, 13.8424) -> (6.6425, 14.1655)
  line L262 (6.7672, 13.5288) -> (6.4479, 13.1206)
  line L263 (6.4413, 12.5973) -> (7.335, 12.5009)
  line L264 (6.8116, 13.6091) -> (6.7672, 13.5288)
  line L265 (6.8569, 13.6913) -> (6.8116, 13.6091)
  line L266 (6.8144, 6.1221) -> (6.3761, 6.569)
  line L267 (7.1451, 6.278) -> (7.1621, 6.2666)
  line L268 (6.9977, 6.3885) -> (7.1451, 6.278)
  line L269 (7.1621, 6.2666) -> (7.267, 6.192)
  line L270 (7.267, 6.192) -> (7.2764, 6.329)
  line L271 (7.2764, 6.329) -> (7.2906, 6.5907)
  line L272 (7.2906, 6.5907) -> (7.2934, 6.653)
  line L273 (7.2934, 6.653) -> (7.2972, 6.7163)
  line L274 (7.2972, 6.7163) -> (7.3123, 6.979)
  line L275 (6.4545, 7.0149) -> (6.9977, 6.3885)
  line L276 (7.0128, 14.6974) -> (6.8191, 14.6917)
  line L277 (6.8191, 14.6634) -> (6.8579, 14.5973)
  line L278 (6.8191, 14.6917) -> (6.8191, 14.6634)
  line L279 (7.335, 12.5009) -> (8.121, 12.0701)
  line L280 (8.121, 12.0701) -> (8.2495, 11.9369)
  line L281 (8.2495, 11.9369) -> (8.3298, 11.8538)
  line L282 (8.8192, 9.9397) -> (8.5253, 9.2473)
  line L283 (8.8437, 10.0947) -> (8.8192, 9.9397)
  line L284 (8.8503, 10.1334) -> (8.8437, 10.0947)
  line L285 (8.8626, 10.4178) -> (8.8503, 10.1334)
  line L286 (8.8503, 10.7021) -> (8.8626, 10.4178)
  line L287 (8.8437, 10.7399) -> (8.8503, 10.7021)
  line L288 (8.8248, 10.8561) -> (8.8437, 10.7399)
  line L289 (8.3298, 11.8538) -> (8.6387, 11.388)
  line L290 (8.6387, 11.388) -> (8.8248, 10.8561)
  line L291 (9.5532, 12.3998) -> (9.7403, 12.6133)
  line L292 (9.7403, 12.6133) -> (9.7894, 12.6681)
  line L293 (9.7894, 12.6681) -> (10.1181, 13.0328)
  line L294 (10.1181, 13.0328) -> (9.2906, 13.8604)
  line L295 (8.7322, 13.3568) -> (8.7105, 13.3379)
  line L296 (8.5584, 13.2009) -> (8.5036, 13.2368)
  line L297 (8.5036, 13.2368) -> (8.4809, 13.2529)
  line L298 (8.7105, 13.3379) -> (8.5584, 13.2009)
  line L299 (9.0771, 13.6676) -> (9.0478, 13.6412)
  line L300 (9.2906, 13.8604) -> (9.0771, 13.6676)
  line L301 (9.0478, 13.6412) -> (8.7322, 13.3568)
  line L302 (8.4809, 13.2529) -> (8.291, 13.3634)
  line L303 (8.291, 13.3634) -> (8.087, 13.4674)
  line L304 (8.5253, 9.2473) -> (8.0237, 8.6889)
  line L305 (8.5348, 7.6167) -> (8.5641, 7.6356)
  line L306 (8.4583, 7.5656) -> (8.5348, 7.6167)
  line L307 (8.0237, 8.6889) -> (7.8943, 8.6011)
  line L308 (7.8943, 8.6011) -> (7.8612, 8.5784)
  line L309 (7.8612, 8.5784) -> (7.6354, 8.4556)
  line L310 (7.6354, 8.4556) -> (7.403, 8.3536)
  line L311 (7.403, 8.3536) -> (7.3652, 8.3413)
  line L312 (7.4569, 7.1509) -> (7.5532, 7.1745)
  line L313 (7.4389, 7.1471) -> (7.4569, 7.1509)
  line L314 (7.3218, 7.115) -> (7.4389, 7.1471)
  line L315 (7.3123, 6.979) -> (7.3218, 7.115)
  line L316 (7.5532, 7.1745) -> (8.4583, 7.5656)
  line L317 (10.8069, 11.0139) -> (10.3808, 11.0366)
  line L318 (10.3808, 11.0366) -> (10.3317, 11.0385)
  line L319 (10.3317, 11.0385) -> (9.9783, 11.0573)
  line L320 (9.7818, 9.1301) -> (9.949, 9.6431)
  line L321 (9.9727, 9.7508) -> (10.0284, 9.7867)
  line L322 (10.0284, 9.7867) -> (10.2995, 9.8037)
  line L323 (10.2995, 9.8037) -> (10.3893, 9.8075)
  line L324 (10.3893, 9.8075) -> (10.4365, 9.8103)
  line L325 (10.4365, 9.8103) -> (10.8154, 9.8302)
  line L326 (10.8154, 9.8302) -> (10.9278, 9.8377)
  line L327 (10.9278, 9.8377) -> (10.9278, 11.0073)
  line L328 (10.9278, 11.0073) -> (10.8069, 11.0139)
  line L329 (9.949, 9.6431) -> (9.9727, 9.7508)
  line L330 (8.5641, 7.6356) -> (8.9287, 7.3068)
  line L331 (8.9287, 7.3068) -> (9.2943, 6.978)
  line L332 (9.2943, 6.978) -> (9.7081, 7.3909)
  line L333 (9.4748, 8.534) -> (9.5078, 8.6039)
  line L334 (9.5721, 8.4206) -> (9.4748, 8.534)
  line L335 (9.5078, 8.6039) -> (9.5636, 8.6861)
  line L336 (9.7554, 8.2128) -> (9.5721, 8.4206)
  line L337 (9.5636, 8.6861) -> (9.7818, 9.1301)
  line L338 (10.1229, 7.8047) -> (9.7998, 8.1627)
  line L339 (9.7081, 7.3909) -> (10.1229, 7.8047)
  line L340 (9.7998, 8.1627) -> (9.7554, 8.2128)
  line L341 (6.3761, 6.569) -> (6.0426, 7.0942)
  line L342 (5.2764, 6.6172) -> (5.4984, 6.4934)
  line L343 (5.4984, 6.4934) -> (5.574, 6.4518)
  line L344 (5.574, 6.4518) -> (6.4167, 6.1183)
  point P0 (6.3, 180)
  point P1 (0.9647, 14.875)
  constraints: 690 end point
emboss "Gravure1" sketch "Esquisse2" operation cut depth 0.05 direction (0, -1, 0)
pattern_linear "Réseau rectangulaire1" count 7 spacing 56 along (0, 0, -1) of "Gravure1"
